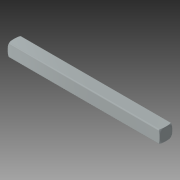
# Autodesk Inventor part: 276-3522
Saved by Autodesk Inventor 2016 SP2 (Build 200236200, 236)
## iProperties
Created: 2016-05-15
Part Number: 276-3522
Material: Generic
Document SubType Name: Modeling
Designer: Jacob
Density: 1 g/cm^3
Appearance: Zinc
Author: Jacob (7842)
Autodesk Inventor part; units mm, degrees
ref_plane "YZ Plane" through (0, 0, 0) normal (1, 0, 0) x (0, 1, 0)
sketch "Sketch1" plane through (0, 0, 0) normal (0, 1, 0) x (-1, 0, 0)
  line L0 (0.508, 0) -> (5.842, 0)
  line L1 (6.35, -0.508) -> (6.35, -5.842)
  line L2 (5.842, -6.35) -> (0.508, -6.35)
  line L3 (0, -5.842) -> (0, -0.508)
  arc A0 (5.842, -6.35) -> (6.35, -5.842) centre (5.842, -5.842) ccw
  arc A1 (0, -5.842) -> (0.508, -6.35) centre (0.508, -5.842) ccw
  arc A2 (0.508, 0) -> (0, -0.508) centre (0.508, -0.508) ccw
  arc A3 (6.35, -0.508) -> (5.842, 0) centre (5.842, -0.508) ccw
  arc A4 (3.874769, -6.35) -> (6.35, -3.874769) centre (3.175, -3.175) ccw
  arc A5 (0, -3.874769) -> (2.475231, -6.35) centre (3.175, -3.175) ccw
  arc A6 (6.35, -2.475231) -> (3.874769, 0) centre (3.175, -3.175) ccw
  arc A7 (2.475231, 0) -> (0, -2.475231) centre (3.175, -3.175) ccw
  point P0 (0, 0)
  point P1 (6.35, -6.35)
  point P2 (6.35, 0)
  point P3 (0, -6.35)
  dimension "d0" = 6.35
  dimension "d1" = 6.35
  dimension "d2" = 0.508
  constraints: 16 point on circle, 16 point on line, 8 centre point, 8 end point, 8 tangent, 3 equal radius, 2 parallel, 1 horizontal, 1 perpendicular
  measures "d0" distance of point (6.35, -6.35) point (0, -6.35)
  measures "d1" distance of point (6.35, 0) point (6.35, -6.35)
  measures "d2" radius of A0
extrude "Extrusion1" add sketch "Sketch1" along normal blind 76.2
ref_plane "Work Plane1" through (-0.508, 0, -3.175) normal (0, 0, -1) x (-1, 0, 0)
sketch "Sketch2" plane through (-0.508, 0, -3.175) normal (0, 0, -1) x (-1, 0, 0)
  line L0 (-0.508, 0) -> (-0.508, 76.2)
  line L1 (-0.508, 76.2) -> (5.842, 76.2)
  line L2 (5.842, 76.2) -> (5.842, 0)
  line L3 (5.842, 0) -> (-0.508, 0)
  line L4 (2.667, 76.2) -> (2.667, 76.9112)
  line L5 (2.667, 76.9112) -> (6.9342, 76.9112)
  line L6 (2.667, 76.2) -> (5.461, 76.2)
  arc A0 (6.9342, 75.692) -> (5.461, 76.2) centre (5.51465, 73.965444) ccw
  line L7 (6.9342, 76.9112) -> (7.192755, 76.9112)
  line L8 (7.192755, 76.9112) -> (7.192755, 75.441954)
  line L9 (7.192755, 75.441954) -> (6.9342, 75.692)
  dimension "d6" = 0.7112
  dimension "d7" = 4.2672
  dimension "d8" = 1.2192
  dimension "d9" = 2.794
  dimension "d10" = 2.2352
  constraints: 12 end point, 2 perpendicular, 2 point on circle, 1 centre point, 1 horizontal, 1 midpoint, 1 point on line, 1 vertical
  measures "d6" distance of L4.start L4.end
  measures "d7" distance of L4.end L5.end
  measures "d8" distance of L5.end L9.end
  measures "d9" distance of L4.start L6.end
  measures "d10" radius of A0
sketch "Sketch2 outline for Revolution1" plane through (-0.508, 0, -3.175) normal (0, 0, -1) x (-1, 0, 0)
  line L0 (2.667, 76.2) -> (5.461, 76.2)
  line L1 (2.667, 76.9112) -> (2.667, 76.2)
  line L2 (6.9342, 76.9112) -> (2.667, 76.9112)
  line L3 (7.192755, 76.9112) -> (6.9342, 76.9112)
  line L4 (7.192755, 75.441954) -> (7.192755, 76.9112)
  line L5 (6.9342, 75.692) -> (7.192755, 75.441954)
  arc A0 (5.461, 76.2) -> (6.9342, 75.692) centre (5.51465, 73.965444) cw
revolve "Revolution1" cut sketch "Sketch2 outline for Revolution1" angle 360 about axis through (-3.175, 76.2, -3.175) along (0, 1, 0)
ref_plane "Work Plane2" through (-3.175, 38.1, -3.175) normal (0, 1, 0) x (1, 0, 0)
mirror "Mirror1" about plane through (-3.175, 38.1, -3.175) normal (0, 1, 0) of "Revolution1"
body "Solid1"
